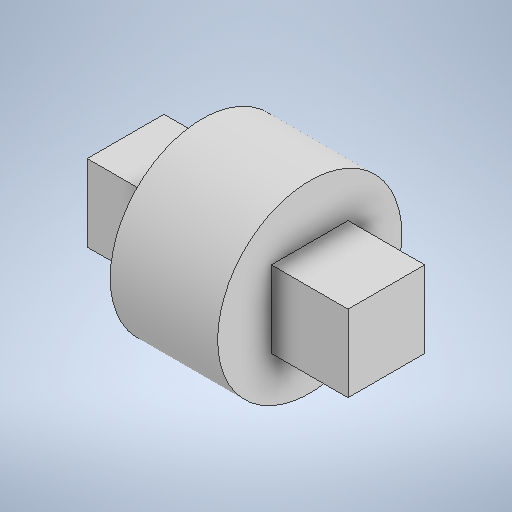
# Autodesk Inventor part: 210 part 3
Saved by Autodesk Inventor 2025.1 (Build 291241000, 241)
## iProperties
Created: 2024-09-02
Part Number: 210 part 3
Material: Generisch
Document SubType Name: Modeling
Designer: ffogue
Density: 1 g/cm^3
Appearance: Vorgabe
Author: ffogue
Autodesk Inventor part; units mm, degrees
ref_plane "XZ Plane" through (0, 0, 0) normal (0, 1, 0) x (-1, 0, 0)
ref_plane "XY Plane" through (0, 0, 0) normal (0, 0, 1) x (1, 0, 0)
sketch "Sketch1" plane through (0, 0, 0) normal (0, 0, 1) x (1, 0, 0)
  line L0 (0, 0) -> (0, 6)
  line L1 (0, 6) -> (7, 6)
  line L2 (7, 6) -> (7, 0)
  line L3 (7, 0) -> (0, 0)
  dimension "d0" = 12
  dimension "d1" = 7
  constraints: 8 end point, 3 perpendicular, 1 vertical
  measures "d0" diameter of L1 L3
  measures "d1" distance of L0.end L1.end
revolve "Revolution1" add sketch "Sketch1" angle 360 about axis through (7, 0, 0) along (-1, 0, 0)
ref_plane "Work Plane1" through (3.5, 0, 0) normal (1, 0, 0) x (0, 1, 0)
sketch "Sketch2" plane through (3.5, 0, 0) normal (1, 0, 0) x (0, 1, 0)
  line L0 (-2.5, 2.5) -> (2.5, 2.5)
  line L1 (2.5, 2.5) -> (2.5, -2.5)
  line L2 (2.5, -2.5) -> (-2.5, -2.5)
  line L3 (-2.5, -2.5) -> (-2.5, 2.5)
  line L4 (-2.5, 2.5) -> (2.5, -2.5) construction
  line L5 (2.5, 2.5) -> (-2.5, -2.5) construction
  point P0 (0, 0)
  dimension "d3" = 5
  dimension "d4" = 5
  constraints: 12 end point, 2 midpoint, 2 parallel, 1 horizontal, 1 perpendicular
  measures "d3" distance of L1.end L2.end
  measures "d4" distance of L0.end L1.end
extrude "Extrusion1" add sketch "Sketch2" along normal mid plane 17
body "Solid1"
